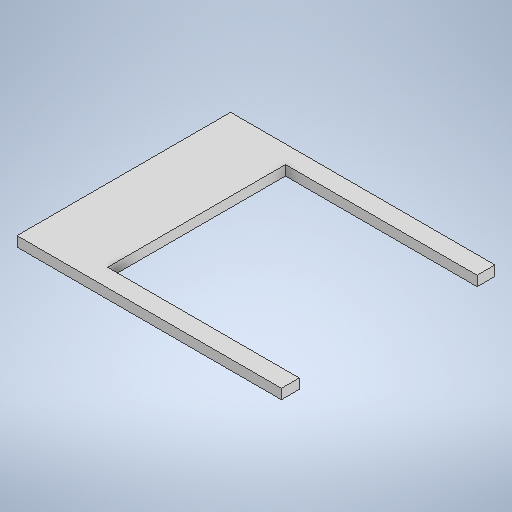
# Autodesk Inventor part: Carcasa_llanta_posible
Saved by Autodesk Inventor 2025.3 (Build 293356030, 356C)
## iProperties
Created: 2025-08-28
Part Number: Carcasa_llanta_posible
Material: Generic
Document SubType Name: Modeling
Designer: brene
Density: 1 g/cm^3
Appearance: Default
Author: brene
Autodesk Inventor part; units mm, degrees
ref_plane "YZ Plane" through (0, 0, 0) normal (1, 0, 0) x (0, 1, 0)
ref_plane "XZ Plane" through (0, 0, 0) normal (0, 1, 0) x (-1, 0, 0)
ref_plane "XY Plane" through (0, 0, 0) normal (0, 0, 1) x (1, 0, 0)
sketch "Sketch1" plane through (0, 0, 0) normal (0, 1, 0) x (-1, 0, 0)
  line L0 (0, 0) -> (80, 0)
  line L1 (80, 0) -> (80, -64.6309)
  line L2 (80, -64.6309) -> (0, -64.6309)
  line L3 (0, -64.6309) -> (0, -59.2309)
  line L4 (0, -59.2309) -> (58, -59.2309)
  line L5 (0, 0) -> (0, -5.4)
  line L6 (0, -5.4) -> (58, -5.4)
  line L7 (58, -5.4) -> (58, -59.2309)
  line L8 (0, -5.4) -> (0, -59.2309)
  dimension "d0" = 80
  dimension "d1" = 64.6308
  dimension "d2" = 5.4
  dimension "d4" = 58
  dimension "d5" = 5.4
  constraints: 18 end point, 4 vertical, 2 horizontal, 2 perpendicular, 1 parallel
  measures "d0" distance of L0.start L0.end
  measures "d1" distance of L0.end L1.end
  measures "d2" distance of L2.end L3.end
  measures "d4" distance of L3.end L4.end
  measures "d5" distance of L0.start L5.end
extrude "Extrusion1" add sketch "Sketch1" along normal blind 3 contours L0 L1 L2 L3 L4 L7 L6 L5
body "Solid1"
